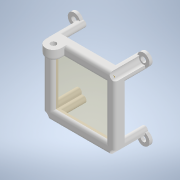
# Autodesk Inventor part: Back
Saved by Autodesk Inventor 2021 (Build 250183000, 183)
## iProperties
Created: 2020-10-20
Part Number: Back
Material: Generic
Document SubType Name: Modeling
Designer: VM
Density: 1 g/cm^3
Appearance: Default
Author: VM
Autodesk Inventor part; units mm, degrees
ref_plane "YZ Plane" through (0, 0, 0) normal (1, 0, 0) x (0, 1, 0)
ref_plane "XZ Plane" through (0, 0, 0) normal (0, 1, 0) x (-1, 0, 0)
ref_plane "XY Plane" through (0, 0, 0) normal (0, 0, 1) x (1, 0, 0)
ref_plane "Work Plane1" through (0, 0, 0) normal (0, 0, 1) x (1, 0, 0)
sketch "Sketch1" plane through (0, 0, 0) normal (0, 0, 1) x (1, 0, 0)
  line L0 (18.9, -18.65) -> (-18.9, -18.65) projected
  line L1 (18.9, 18.65) -> (18.9, -18.65) projected
  line L2 (-18.9, 18.65) -> (18.9, 18.65) projected
  line L3 (-18.9, -18.65) -> (-18.9, 18.65) projected
  line L4 (19.3, 19.05) -> (19.3, -19.05)
  line L5 (19.3, -19.05) -> (-19.3, -19.05)
  line L6 (-19.3, -19.05) -> (-19.3, 19.05)
  line L7 (-19.3, 19.05) -> (19.3, 19.05)
  line L8 (23.3, 23.05) -> (23.3, -23.05)
  line L9 (23.3, -23.05) -> (-23.3, -23.05)
  line L10 (-23.3, -23.05) -> (-23.3, 23.05)
  line L11 (-23.3, 23.05) -> (23.3, 23.05)
  point P0 (0, 0)
  dimension "d0" = 0.4
  dimension "d1" = 4
  constraints: 16 end point, 6 other
  measures "d0" distance between parallel lines of L2 L7
  measures "d1" distance between parallel lines of L7 L11
extrude "Extrusion1" add sketch "Sketch1" against normal blind 4 contours L8 L9 L10 L11
sketch "Sketch2" plane through (0, 0, 0) normal (0, 0, 1) x (1, 0, 0)
  line L0 (18.9, -18.65) -> (-18.9, -18.65) projected
  line L1 (18.9, 18.65) -> (18.9, -18.65) projected
  line L2 (-18.9, 18.65) -> (18.9, 18.65) projected
  line L3 (-18.9, -18.65) -> (-18.9, 18.65) projected
  line L4 (16.9, 16.65) -> (16.9, -16.65)
  line L5 (16.9, -16.65) -> (-16.9, -16.65)
  line L6 (-16.9, -16.65) -> (-16.9, 16.65)
  line L7 (-16.9, 16.65) -> (16.9, 16.65)
  line L8 (23.3, 23.05) -> (23.3, -23.05)
  line L9 (23.3, -23.05) -> (-23.3, -23.05)
  line L10 (-23.3, -23.05) -> (-23.3, 23.05)
  line L11 (-23.3, 23.05) -> (23.3, 23.05)
  point P0 (0, 0)
  dimension "d4" = 2
  constraints: 16 end point, 6 other
  measures "d4" distance between parallel lines of L2 L7
extrude "Extrusion2" add sketch "Sketch2" along normal blind 2 contours L0 L3 L2 L1 | L8 L9 L10 L11
sketch "Sketch3" plane through (0, 0, -4) normal (0, 0, -1) x (-1, 0, 0)
  line L0 (-19.3, -19.05) -> (-19.3, 19.05) projected
  line L1 (-19.3, 19.05) -> (-16.2619, 19.05)
  line L2 (-16.2619, 19.05) -> (-16.2619, 23.05)
  line L3 (23.3, 23.05) -> (-23.3, 23.05) projected
  line L4 (-19.3, 19.05) -> (-19.3, 16.0244)
  line L5 (-19.3, 16.0244) -> (-23.3, 16.0244)
  line L6 (-23.3, 23.05) -> (-23.3, -23.05) projected
  circle A0 centre (-22.3, 22.05) radius 2.75
  line L7 (0, 23.05) -> (0, -23.05)
  line L8 (-23.3, -23.05) -> (23.3, -23.05) projected
  line L9 (-23.3, 0) -> (23.3, 0)
  line L10 (19.3, 19.05) -> (16.2619, 19.05)
  line L11 (16.2619, 19.05) -> (16.2619, 23.05)
  line L12 (19.3, 19.05) -> (19.3, 16.0244)
  line L13 (19.3, 16.0244) -> (23.3, 16.0244)
  circle A1 centre (22.3, 22.05) radius 2.75
  line L14 (-19.3, -19.05) -> (-16.2619, -19.05)
  line L15 (-16.2619, -19.05) -> (-16.2619, -23.05)
  line L16 (23.3, -23.05) -> (-23.3, -23.05)
  line L17 (-19.3, -19.05) -> (-19.3, -16.0244)
  line L18 (-19.3, -16.0244) -> (-23.3, -16.0244)
  circle A2 centre (-22.3, -22.05) radius 2.75
  line L19 (19.3, -19.05) -> (16.2619, -19.05)
  line L20 (16.2619, -19.05) -> (16.2619, -23.05)
  line L21 (19.3, -19.05) -> (19.3, -16.0244)
  line L22 (19.3, -16.0244) -> (23.3, -16.0244)
  circle A3 centre (22.3, -22.05) radius 2.75
  line L23 (23.3, -23.05) -> (23.3, 23.05) projected
  line L24 (23.3, 23.05) -> (-23.3, 23.05) projected
  line L25 (-23.3, 23.05) -> (-23.3, -23.05) projected
  line L26 (-23.3, -23.05) -> (23.3, -23.05) projected
  line L27 (-19.3, -19.05) -> (-19.3, 19.05) projected
  line L28 (-19.3, 19.05) -> (19.3, 19.05) projected
  line L29 (19.3, 19.05) -> (19.3, -19.05) projected
  line L30 (19.3, -19.05) -> (-19.3, -19.05) projected
  point P0 (0, 0)
  point P1 (-19.7383, 23.05)
  point P2 (-23.3, 19.4883)
  point P3 (-23.3, -19.4883)
  point P4 (-19.7383, -23.05)
  point P5 (23.3, -19.4883)
  point P6 (19.7383, -23.05)
  point P7 (23.3, 19.4883)
  point P8 (19.7383, 23.05)
  dimension "d7" = 5.5
  dimension "d8" = 1
  dimension "d9" = 1
  constraints: 38 end point, 17 symmetric about line, 4 centre point, 3 midpoint, 3 point on line, 2 horizontal, 2 perpendicular, 1 vertical, 3 other
  measures "d7" diameter of A0
  measures "d8" horizontal distance of L3.end A0.centre
  measures "d9" distance from line of L3 A0.centre
extrude "Extrusion3" add sketch "Sketch3" along normal blind 15 contours L14 L15 L8 A2 L6 L18 L0 | L5 L6 A0 L3 L2 L1 L0 | L19 L21 L22 L23 A3 L8 L20 | L11 L3 A1 L23 L13 L12 L10
sketch "Sketch4" plane through (0, 0, -4) normal (0, 0, -1) x (-1, 0, 0)
  arc A0 (-23.3, 19.4883) -> (-19.7383, 23.05) centre (-22.3, 22.05) ccw projected
  line L0 (-19.7383, 23.05) -> (-23.3, 23.05) projected
  line L1 (-23.3, 23.05) -> (-23.3, 19.4883) projected
  arc A1 (19.7383, 23.05) -> (23.3, 19.4883) centre (22.3, 22.05) ccw projected
  line L2 (23.3, 19.4883) -> (23.3, 23.05) projected
  line L3 (23.3, 23.05) -> (19.7383, 23.05) projected
  arc A2 (23.3, -19.4883) -> (19.7383, -23.05) centre (22.3, -22.05) ccw projected
  line L4 (19.7383, -23.05) -> (23.3, -23.05) projected
  line L5 (23.3, -23.05) -> (23.3, -19.4883) projected
  arc A3 (-19.7383, -23.05) -> (-23.3, -19.4883) centre (-22.3, -22.05) ccw projected
  line L6 (-23.3, -19.4883) -> (-23.3, -23.05) projected
  line L7 (-23.3, -23.05) -> (-19.7383, -23.05) projected
  point P0 (0, 0)
extrude "Extrusion4" cut sketch "Sketch4" against normal blind 19
sketch "Sketch5" plane through (0, 0, -19) normal (0, 0, -1) x (-1, 0, 0)
  circle A0 centre (22.3, 22.05) radius 1.75
  arc A1 (19.7383, 23.05) -> (23.3, 19.4883) centre (22.3, 22.05) ccw projected
  circle A2 centre (22.3, 22.05) radius 4
  line L0 (23.3, -16.0244) -> (23.3, 16.0244) projected
  line L1 (23.3, 0) -> (-23.3, 0)
  line L2 (-23.3, 16.0244) -> (-23.3, -16.0244) projected
  line L3 (16.2619, 23.05) -> (-16.2619, 23.05) projected
  line L4 (0, 23.05) -> (0, -23.05)
  line L5 (-16.2619, -23.05) -> (16.2619, -23.05) projected
  circle A3 centre (22.3, -22.05) radius 1.75
  arc A4 (23.3, -19.4883) -> (19.7383, -23.05) centre (22.3, -22.05) ccw
  circle A5 centre (22.3, -22.05) radius 4
  circle A6 centre (-22.3, 22.05) radius 1.75
  arc A7 (-23.3, 19.4883) -> (-19.7383, 23.05) centre (-22.3, 22.05) ccw
  circle A8 centre (-22.3, 22.05) radius 4
  line L6 (-23.3, -16.0244) -> (-23.3, 16.0244)
  circle A9 centre (-22.3, -22.05) radius 1.75
  arc A10 (-19.7383, -23.05) -> (-23.3, -19.4883) centre (-22.3, -22.05) ccw
  circle A11 centre (-22.3, -22.05) radius 4
  point P0 (0, 0)
  dimension "d14" = 3.5
  dimension "d15" = 8
  constraints: 15 symmetric about line, 11 centre point, 6 end point, 6 point on circle, 4 coincident, 4 midpoint, 1 concentric, 9 other
  measures "d14" diameter of A0
  measures "d15" diameter of A2
extrude "Extrusion5" add sketch "Sketch5" against normal blind 2
fillet "Fillet1" radius 2 16 edges at (-16.2619, 19.05, -11.5) (-19.3, 16.0244, -11.5) (-16.2619, -23.05, -11.5) (-16.2619, -19.05, -11.5) (-19.3, -16.0244, -11.5) (-23.3, -16.0244, -11.5) (-16.2619, 23.05, -11.5) (-23.3, 16.0244, -11.5) (23.3, 16.0244, -11.5) (19.3, 16.0244, -11.5) (16.2619, 19.05, -11.5) (16.2619, 23.05, -11.5) (23.3, -16.0244, -11.5) (19.3, -16.0244, -11.5) (16.2619, -19.05, -11.5) (16.2619, -23.05, -11.5)
sketch "Sketch6" plane through (0, 0, 2) normal (0, 0, 1) x (1, 0, 0)
  line L0 (-19.55, 23.05) -> (-9.55, 23.05)
  line L1 (-9.55, 23.05) -> (-9.55, 16.65)
  line L2 (-9.55, 16.65) -> (-19.55, 16.65)
  line L3 (-19.55, 16.65) -> (-19.55, 23.05)
  arc A0 (-23.3, 19.4883) -> (-19.7383, 23.05) centre (-22.3, 22.05) ccw projected
  line L4 (-16.9, 16.65) -> (16.9, 16.65) projected
  point P0 (0, 0)
  dimension "d19" = 10
  dimension "d20" = 6.4
  constraints: 8 end point, 2 parallel, 1 collinear, 1 horizontal, 1 perpendicular, 1 tangent
  measures "d19" distance of L1.end L2.end
  measures "d20" distance of L0.end L1.end
extrude "Extrusion6" add sketch "Sketch6" along normal blind 7
fillet "Fillet2" radius 5 2 edges at (-19.55, 19.85, 9) (-9.55, 19.85, 9)
sketch "Sketch7" plane through (-16.9, 16.65, 0) normal (0, -1, 0) x (1, 0, 0)
  arc A0 (7.35, 4) -> (-2.65, 4) centre (2.35, 4) ccw projected
  point P0 (16.9, 0)
  constraints: 1 coincident
hole "Hole1" at (-14.55, 16.65, 4) direction (0, 1, 0) diameter 3.5 end through all counterbore diameter 5.6 counterbore depth 2.4
fillet "Fillet3" radius 2 8 edges at (0, -23.05, 2) (-23.3, 0, 2) (5.0941, 23.05, 2) (23.3, 0, 2) (-16.9, 0, 2) (0, -16.65, 2) (3.675, 16.65, 2) (16.9, 0, 2)
fillet "Fillet4" radius 2 5 edges at (-9.55, 16.65, 2.0001) (-19.55, 16.65, 3.0001) (-18.0856, 16.65, 7.5356) (-14.55, 16.65, 9) (-11.0144, 16.65, 7.5356)
body "Solid1"
